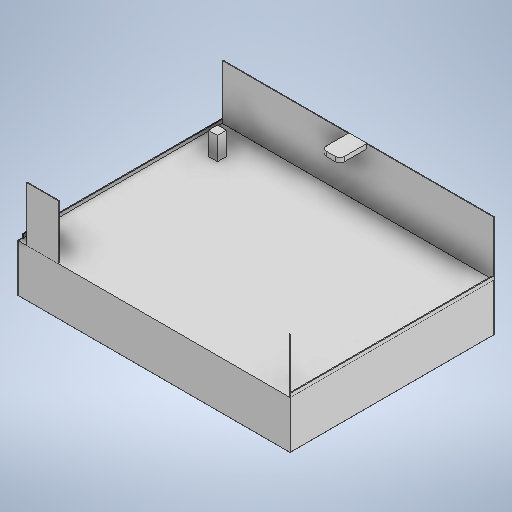
# Autodesk Inventor part: game base
Saved by Autodesk Inventor 2025.4 (Build 294407000, 407)
## iProperties
Created: 2026-03-10
Part Number: game base
Material: Generic
Document SubType Name: Modeling
Designer: youse
Density: 1 g/cm^3
Appearance: Default
Author: youse
Autodesk Inventor part; units mm, degrees
ref_plane "YZ Plane" through (0, 0, 0) normal (1, 0, 0) x (0, 1, 0)
ref_plane "XZ Plane" through (0, 0, 0) normal (0, 1, 0) x (-1, 0, 0)
ref_plane "XY Plane" through (0, 0, 0) normal (0, 0, 1) x (1, 0, 0)
sketch "Sketch1" plane through (0, 0, 0) normal (0, 1, 0) x (-1, 0, 0)
  line L0 (-300, 225) -> (300, 225)
  line L1 (300, 225) -> (300, -225)
  line L2 (300, -225) -> (-300, -225)
  line L3 (-300, -225) -> (-300, 225)
  line L4 (-300, 225) -> (300, -225) construction
  line L5 (300, 225) -> (-300, -225) construction
  point P0 (0, 0)
  dimension "d0" = 600
  dimension "d1" = 450
  constraints: 12 end point, 2 midpoint, 2 parallel, 1 horizontal, 1 perpendicular
  measures "d0" distance of L1.end L2.end
  measures "d1" distance of L0.end L1.end
extrude "Extrusion1" add sketch "Sketch1" along normal blind 5
sketch "Sketch6" plane through (0, 5, 0) normal (0, 1, 0) x (1, 0, 0)
  line L0 (300, 225) -> (-300, 225) projected
  line L1 (-300, -225) -> (300, -225)
  line L2 (300, -225) -> (300, 225)
  line L3 (300, 225) -> (-300, 225)
  line L4 (-300, 225) -> (-300, -225)
  line L5 (-300, -225) -> (300, 225) construction
  line L6 (300, -225) -> (-300, 225) construction
  line L7 (-298, -223.5) -> (298, -223.5)
  line L8 (298, -223.5) -> (298, 223.5)
  line L9 (298, 223.5) -> (-298, 223.5)
  line L10 (-298, 223.5) -> (-298, -223.5)
  line L11 (-298, -223.5) -> (298, 223.5) construction
  line L12 (298, -223.5) -> (-298, 223.5) construction
  point P0 (0, 0)
  dimension "d26" = 2
  constraints: 24 end point, 4 midpoint, 4 parallel, 2 horizontal, 2 perpendicular, 1 point on line
  measures "d26" distance between parallel lines of L2 L8
extrude "Extrusion7" add sketch "Sketch6" along normal blind 120
sketch "Sketch7" plane through (0, 0, 0) normal (0, -1, 0) x (1, 0, 0)
  line L0 (300, 225) -> (300, -225) projected
  line L1 (-300, 225) -> (300, 225)
  line L2 (300, 225) -> (300, -225)
  line L3 (300, -225) -> (-300, -225)
  line L4 (-300, -225) -> (-300, 225)
  line L5 (-300, 225) -> (300, -225) construction
  line L6 (300, 225) -> (-300, -225) construction
  point P0 (0, 0)
  constraints: 12 end point, 2 midpoint, 2 parallel, 1 horizontal, 1 perpendicular
extrude "Extrusion8" add sketch "Sketch7" along normal blind 100
shell "Shell1" thickness 1 removed faces 1 at (-100, -100, 75)
mirror "Mirror1" about plane through (0, 0, 0) normal (0, 0, 1)
sketch "Sketch9" plane through (0, 125, 0) normal (0, 1, 0) x (1, 0, 0)
  line L0 (300, 225) -> (-300, 225) projected
  line L1 (-20, 225) -> (20, 225)
  line L2 (20, 225) -> (20, 175)
  line L3 (10, 165) -> (-10, 165)
  line L4 (-20, 175) -> (-20, 225)
  arc A0 (-20, 175) -> (-10, 165) centre (-10, 175) ccw
  arc A1 (10, 165) -> (20, 175) centre (10, 175) ccw
  point P0 (0, 0)
  point P1 (20, 165)
  point P2 (-20, 165)
  point P3 (0, 225)
  dimension "d37" = 40
  dimension "d38" = 60
  dimension "d39" = 10
  constraints: 8 end point, 5 point on line, 4 point on circle, 4 tangent, 2 centre point, 2 midpoint, 2 parallel, 1 equal radius, 1 horizontal, 1 perpendicular
  measures "d37" distance of point (20, 165) point (-20, 165)
  measures "d38" distance between parallel lines of L0 L3
  measures "d39" radius of A0
extrude "Extrusion10" add sketch "Sketch9" against normal blind 10
sketch "Sketch10" plane through (0, 5, 0) normal (0, 1, 0) x (1, 0, 0)
  line L0 (-230, 165) -> (-250, 165)
  line L1 (-250, 165) -> (-250, 145)
  line L2 (-250, 145) -> (-230, 145)
  line L3 (-230, 145) -> (-230, 165)
  line L4 (-300, 225) -> (-300, -225) projected
  line L5 (300, 225) -> (-300, 225) projected
  point P0 (0, 0)
  point P1 (-250, 155)
  point P2 (-240, 165)
  dimension "d42" = 20
  dimension "d43" = 20
  dimension "d44" = 50
  dimension "d45" = 60
  constraints: 8 end point, 2 midpoint, 2 parallel, 1 horizontal, 1 perpendicular
  measures "d42" distance of L2.end L0.start
  measures "d43" distance of L1.end L2.end
  measures "d44" distance from line of L4 point (-250, 155)
  measures "d45" distance from line of L5 point (-240, 165)
extrude "Extrusion11" add sketch "Sketch10" along normal blind 50
sketch "Sketch11" plane through (-298, 5, 223.5) normal (1, 0, 0) x (0, 0, -1)
  line L0 (448.5, 120) -> (448.5, -105) projected
  line L1 (0, 120) -> (448.5, 120)
  line L2 (448.5, 120) -> (448.5, 7.5)
  line L3 (448.5, 7.5) -> (0, 7.5)
  line L4 (0, 7.5) -> (0, 120)
  point P0 (223.5, -5)
  constraints: 8 end point, 2 parallel, 1 horizontal, 1 midpoint, 1 perpendicular
extrude "Extrusion12" cut sketch "Sketch11" against normal through all
sketch "Sketch12" plane through (300, 125, 225) normal (1, 0, 0) x (0, 0, -1)
  line L0 (1.5, 0) -> (1.5, -112.5) projected
  line L1 (448.5, -120) -> (448.5, -112.5) projected
  line L2 (1.5, 0) -> (448.5, 0)
  line L3 (448.5, 0) -> (448.5, -112.5)
  line L4 (448.5, -112.5) -> (1.5, -112.5)
  line L5 (1.5, -112.5) -> (1.5, 0)
  point P0 (225, -125)
  constraints: 8 end point, 2 parallel, 1 horizontal, 1 perpendicular
extrude "Extrusion13" cut sketch "Sketch12" against normal blind 10
sketch "Sketch13" plane through (-300, 125, 225) normal (0, 0, 1) x (1, 0, 0)
  line L0 (2, 0) -> (280, 0) projected
  line L1 (598, -120) -> (2, -120) projected
  line L2 (90, 0) -> (598, 0)
  line L3 (598, 0) -> (598, -120)
  line L4 (598, -120) -> (90, -120)
  line L5 (90, -120) -> (90, 0)
  line L6 (0, -225) -> (0, 0) projected
  point P0 (300, -125)
  point P1 (90, -120)
  dimension "d52" = 90
  constraints: 8 end point, 2 parallel, 1 horizontal, 1 perpendicular, 1 point on line
  measures "d52" distance between parallel lines of L5 L6
extrude "Extrusion14" cut sketch "Sketch13" against normal blind 10
sketch "Sketch14" plane through (298, 5, 225) normal (0, 0, 1) x (1, 0, 0)
  line L0 (-598, -105) -> (-598, 120) projected
  line L1 (-596, 0) -> (-508, 0) projected
  line L2 (-598, 120) -> (-578, 120)
  line L3 (-578, 120) -> (-578, 0)
  line L4 (-578, 0) -> (-598, 0)
  line L5 (-598, 0) -> (-598, 120)
  point P0 (-298, -5)
  dimension "d55" = 20
  constraints: 8 end point, 2 parallel, 1 horizontal, 1 perpendicular, 1 point on line
  measures "d55" distance between parallel lines of L3 L0
extrude "Extrusion15" cut sketch "Sketch14" against normal blind 10
sketch "Sketch15" plane through (300, -100, -225) normal (0, 0, -1) x (-1, 0, 0)
  point P0 (300, 100)
ref_plane "Work Plane1" through (0, 0, 0) normal (0, 0, 1) x (1, 0, 0)
body "Solid1"
